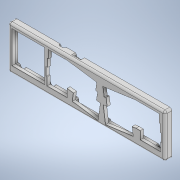
# Autodesk Inventor part: Prime_BLE_Top
Saved by Autodesk Inventor 2020 (Build 240168000, 168)
## iProperties
Created: 2019-06-10
Part Number: Prime_BLE_Top
Material: Generic
Document SubType Name: Modeling
Designer: Holt
Density: 1 g/cm^3
Appearance: Default
Author: Holt
Autodesk Inventor part; units mm, degrees
ref_plane "YZ Plane" through (0, 0, 0) normal (1, 0, 0) x (0, 1, 0)
ref_plane "XZ Plane" through (0, 0, 0) normal (0, 1, 0) x (-1, 0, 0)
ref_plane "XY Plane" through (0, 0, 0) normal (0, 0, 1) x (1, 0, 0)
sketch "Sketch1" plane through (0, 0, 0) normal (0, 0, 1) x (1, 0, 0)
  line L0 (193.827, 71.8136) -> (191.879, 57.9494)
  line L1 (191.879, 57.9494) -> (178.015, 59.8978)
  line L2 (178.015, 59.8978) -> (179.964, 73.7609)
  line L3 (179.964, 73.7609) -> (193.827, 71.8136)
  line L4 (335.021, 71.8149) -> (348.885, 73.7633)
  line L5 (348.885, 73.7633) -> (350.832, 59.8991)
  line L6 (350.832, 59.8991) -> (336.97, 57.9503)
  line L7 (336.97, 57.9503) -> (335.021, 71.8149)
  line L8 (137.682, 59.5644) -> (137.682, 73.5665)
  line L9 (137.682, 73.5665) -> (151.684, 73.5665)
  line L10 (151.684, 73.5665) -> (151.684, 59.5644)
  line L11 (151.684, 59.5644) -> (137.682, 59.5644)
  line L12 (173.018, 59.5644) -> (159.019, 59.5644)
  line L13 (159.019, 59.5644) -> (159.019, 73.5665)
  line L14 (159.019, 73.5665) -> (173.018, 73.5665)
  line L15 (173.018, 73.5665) -> (173.018, 59.5644)
  line L16 (369.901, 73.4147) -> (369.901, 59.4126)
  line L17 (369.901, 59.4126) -> (355.9, 59.4126)
  line L18 (355.9, 59.4126) -> (355.9, 73.4147)
  line L19 (355.9, 73.4147) -> (369.901, 73.4147)
  line L20 (382.093, 59.4126) -> (382.093, 73.4147)
  line L21 (382.093, 73.4147) -> (396.095, 73.4147)
  line L22 (396.095, 73.4147) -> (396.095, 59.4126)
  line L23 (396.095, 59.4126) -> (382.093, 59.4126)
  line L24 (271.059, 82.062) -> (284.924, 84.0118)
  line L25 (284.924, 84.0118) -> (286.872, 70.1473)
  line L26 (286.872, 70.1473) -> (273.008, 68.1989)
  line L27 (273.008, 68.1989) -> (271.059, 82.062)
  line L28 (248.36, 83.3998) -> (246.4211, 69.534)
  line L29 (246.4211, 69.534) -> (232.5558, 71.4724)
  line L30 (232.5558, 71.4724) -> (234.4947, 85.3381)
  line L31 (234.4947, 85.3381) -> (248.36, 83.3998)
  line L32 (291.873, 70.8504) -> (289.925, 84.7135)
  line L33 (289.925, 84.7135) -> (303.788, 86.6619)
  line L34 (303.788, 86.6619) -> (305.736, 72.7988)
  line L35 (305.736, 72.7988) -> (291.873, 70.8504)
  line L36 (227.5465, 72.1776) -> (213.6831, 74.1236)
  line L37 (213.6831, 74.1236) -> (215.6277, 87.9871)
  line L38 (215.6277, 87.9871) -> (229.4921, 86.0411)
  line L39 (229.4921, 86.0411) -> (227.5465, 72.1776)
  line L40 (324.5931, 75.4388) -> (310.7292, 73.498)
  line L41 (310.7292, 73.498) -> (308.7877, 87.3634)
  line L42 (308.7877, 87.3634) -> (322.6526, 89.3043)
  line L43 (322.6526, 89.3043) -> (324.5931, 75.4388)
  line L44 (194.8151, 76.7745) -> (196.7632, 90.6378)
  line L45 (196.7632, 90.6378) -> (210.6263, 88.6898)
  line L46 (210.6263, 88.6898) -> (208.6802, 74.8256)
  line L47 (208.6802, 74.8256) -> (194.8151, 76.7745)
  line L48 (341.5207, 91.9896) -> (343.4929, 78.13)
  line L49 (343.4929, 78.13) -> (329.6334, 76.1573)
  line L50 (329.6334, 76.1573) -> (327.6601, 90.017)
  line L51 (327.6601, 90.017) -> (341.5207, 91.9896)
  line L52 (177.899, 93.2889) -> (191.762, 91.3405)
  line L53 (191.762, 91.3405) -> (189.814, 77.4774)
  line L54 (189.814, 77.4774) -> (175.949, 79.4247)
  line L55 (175.949, 79.4247) -> (177.899, 93.2889)
  line L56 (367.52, 78.6542) -> (367.52, 92.6549)
  line L57 (367.52, 92.6549) -> (381.52, 92.6549)
  line L58 (381.52, 92.6549) -> (381.52, 78.6542)
  line L59 (381.52, 78.6542) -> (367.52, 78.6542)
  line L60 (400.572, 92.6549) -> (400.572, 78.6542)
  line L61 (400.572, 78.6542) -> (386.572, 78.6542)
  line L62 (386.572, 78.6542) -> (386.572, 92.6549)
  line L63 (386.572, 92.6549) -> (400.572, 92.6549)
  line L64 (151.874, 78.8046) -> (137.874, 78.8046)
  line L65 (137.874, 78.8046) -> (137.874, 92.8067)
  line L66 (137.874, 92.8067) -> (151.874, 92.8067)
  line L67 (151.874, 92.8067) -> (151.874, 78.8046)
  line L68 (156.924, 92.8067) -> (170.924, 92.8067)
  line L69 (170.924, 92.8067) -> (170.924, 78.8046)
  line L70 (170.924, 78.8046) -> (156.924, 78.8046)
  line L71 (156.924, 78.8046) -> (156.924, 92.8067)
  line L72 (348.47, 78.6528) -> (348.47, 92.6549)
  line L73 (348.47, 92.6549) -> (362.472, 92.6549)
  line L74 (362.472, 92.6549) -> (362.472, 78.6528)
  line L75 (362.472, 78.6528) -> (348.47, 78.6528)
  line L76 (279.4658, 26.5127) -> (282.7331, 26.9708)
  line L77 (282.7331, 26.9708) -> (282.8681, 26.0103)
  line L78 (282.8681, 26.0103) -> (303.1679, 28.8637)
  line L79 (303.1679, 28.8637) -> (303.033, 29.8243)
  line L80 (303.033, 29.8243) -> (306.3022, 30.2828)
  line L81 (306.3022, 30.2828) -> (306.4372, 29.3223)
  line L82 (306.4372, 29.3223) -> (309.383, 29.737)
  line L83 (309.383, 29.737) -> (311.3317, 15.874)
  line L84 (311.3317, 15.874) -> (278.603, 11.273)
  line L85 (278.603, 11.273) -> (276.6549, 25.1376)
  line L86 (276.6549, 25.1376) -> (279.6011, 25.5509)
  line L87 (279.6011, 25.5509) -> (279.4658, 26.5127)
  line L88 (106.443, 78.8067) -> (106.443, 92.8067)
  line L89 (106.443, 92.8067) -> (120.443, 92.8067)
  line L90 (120.443, 92.8067) -> (120.443, 78.8067)
  line L91 (120.443, 78.8067) -> (106.443, 78.8067)
  line L92 (101.393, 78.8067) -> (87.393, 78.8067)
  line L93 (87.393, 78.8067) -> (87.393, 92.8067)
  line L94 (87.393, 92.8067) -> (101.393, 92.8067)
  line L95 (101.393, 92.8067) -> (101.393, 78.8067)
  line L96 (68.343, 92.8067) -> (82.343, 92.8067)
  line L97 (82.343, 92.8067) -> (82.343, 78.8067)
  line L98 (82.343, 78.8067) -> (68.343, 78.8067)
  line L99 (68.343, 78.8067) -> (68.343, 92.8067)
  line L100 (49.293, 78.8067) -> (49.293, 92.8067)
  line L101 (49.293, 92.8067) -> (63.293, 92.8067)
  line L102 (63.293, 92.8067) -> (63.293, 78.8067)
  line L103 (63.293, 78.8067) -> (49.293, 78.8067)
  line L104 (120.443, 59.7567) -> (106.443, 59.7567)
  line L105 (106.443, 59.7567) -> (106.443, 73.7567)
  line L106 (106.443, 73.7567) -> (120.443, 73.7567)
  line L107 (120.443, 73.7567) -> (120.443, 59.7567)
  line L108 (87.393, 59.7567) -> (87.393, 73.7567)
  line L109 (87.393, 73.7567) -> (101.393, 73.7567)
  line L110 (101.393, 73.7567) -> (101.393, 59.7567)
  line L111 (101.393, 59.7567) -> (87.393, 59.7567)
  line L112 (68.343, 73.7567) -> (82.343, 73.7567)
  line L113 (82.343, 73.7567) -> (82.343, 59.7567)
  line L114 (82.343, 59.7567) -> (68.343, 59.7567)
  line L115 (68.343, 59.7567) -> (68.343, 73.7567)
  line L116 (63.293, 73.7567) -> (63.293, 59.7567)
  line L117 (63.293, 59.7567) -> (49.293, 59.7567)
  line L118 (49.293, 59.7567) -> (49.293, 73.7567)
  line L119 (49.293, 73.7567) -> (63.293, 73.7567)
  line L120 (106.443, 54.7067) -> (120.443, 54.7067)
  line L121 (120.443, 54.7067) -> (120.443, 40.7067)
  line L122 (120.443, 40.7067) -> (106.443, 40.7067)
  line L123 (106.443, 40.7067) -> (106.443, 54.7067)
  line L124 (101.393, 40.7067) -> (87.393, 40.7067)
  line L125 (87.393, 40.7067) -> (87.393, 54.7067)
  line L126 (87.393, 54.7067) -> (101.393, 54.7067)
  line L127 (101.393, 54.7067) -> (101.393, 40.7067)
  line L128 (68.343, 54.7067) -> (82.343, 54.7067)
  line L129 (82.343, 54.7067) -> (82.343, 40.7067)
  line L130 (82.343, 40.7067) -> (68.343, 40.7067)
  line L131 (68.343, 40.7067) -> (68.343, 54.7067)
  line L132 (63.293, 40.7067) -> (49.293, 40.7067)
  line L133 (49.293, 40.7067) -> (49.293, 54.7067)
  line L134 (49.293, 54.7067) -> (63.293, 54.7067)
  line L135 (63.293, 54.7067) -> (63.293, 40.7067)
  line L136 (120.443, 35.6567) -> (120.443, 21.6567)
  line L137 (120.443, 21.6567) -> (106.443, 21.6567)
  line L138 (106.443, 21.6567) -> (106.443, 35.6567)
  line L139 (106.443, 35.6567) -> (120.443, 35.6567)
  line L140 (101.393, 35.6567) -> (101.393, 21.6567)
  line L141 (101.393, 21.6567) -> (87.393, 21.6567)
  line L142 (87.393, 21.6567) -> (87.393, 35.6567)
  line L143 (87.393, 35.6567) -> (101.393, 35.6567)
  line L144 (82.343, 35.6567) -> (82.343, 21.6567)
  line L145 (82.343, 21.6567) -> (68.343, 21.6567)
  line L146 (68.343, 21.6567) -> (68.343, 35.6567)
  line L147 (68.343, 35.6567) -> (82.343, 35.6567)
  line L148 (49.293, 35.6567) -> (63.293, 35.6567)
  line L149 (63.293, 35.6567) -> (63.293, 21.6567)
  line L150 (63.293, 21.6567) -> (49.293, 21.6567)
  line L151 (49.293, 21.6567) -> (49.293, 35.6567)
  line L152 (214.464, 30.4381) -> (212.514, 16.5751)
  line L153 (212.514, 16.5751) -> (198.651, 18.5236)
  line L154 (198.651, 18.5236) -> (200.6, 32.3867)
  line L155 (200.6, 32.3867) -> (214.464, 30.4381)
  line L156 (254.551, 24.8047) -> (252.603, 10.9416)
  line L157 (252.603, 10.9416) -> (219.874, 15.5401)
  line L158 (219.874, 15.5401) -> (221.823, 29.4046)
  line L159 (221.823, 29.4046) -> (224.769, 28.9898)
  line L160 (224.769, 28.9898) -> (224.904, 29.9516)
  line L161 (224.904, 29.9516) -> (228.171, 29.4914)
  line L162 (228.171, 29.4914) -> (228.036, 28.5309)
  line L163 (228.036, 28.5309) -> (248.336, 25.6784)
  line L164 (248.336, 25.6784) -> (248.471, 26.6389)
  line L165 (248.471, 26.6389) -> (251.74, 26.1786)
  line L166 (251.74, 26.1786) -> (251.605, 25.2181)
  line L167 (251.605, 25.2181) -> (254.551, 24.8047)
  line L168 (150.826, 35.0848) -> (150.826, 21.0854)
  line L169 (150.826, 21.0854) -> (136.826, 21.0854)
  line L170 (136.826, 21.0854) -> (136.826, 35.0848)
  line L171 (136.826, 35.0848) -> (150.826, 35.0848)
  line L172 (160.638, 35.0848) -> (174.637, 35.0848)
  line L173 (174.637, 35.0848) -> (174.637, 21.0854)
  line L174 (174.637, 21.0854) -> (160.638, 21.0854)
  line L175 (160.638, 21.0854) -> (160.638, 35.0848)
  line L176 (334.913, 19.1876) -> (321.049, 17.2391)
  line L177 (321.049, 17.2391) -> (319.1, 31.1021)
  line L178 (319.1, 31.1021) -> (332.965, 33.052)
  line L179 (332.965, 33.052) -> (334.913, 19.1876)
  line L180 (387.427, 20.9336) -> (387.427, 34.933)
  line L181 (387.427, 34.933) -> (401.426, 34.933)
  line L182 (401.426, 34.933) -> (401.426, 20.9336)
  line L183 (401.426, 20.9336) -> (387.427, 20.9336)
  line L184 (271.646, 43.6699) -> (285.509, 45.6197)
  line L185 (285.509, 45.6197) -> (287.459, 31.7553)
  line L186 (287.459, 31.7553) -> (273.595, 29.8068)
  line L187 (273.595, 29.8068) -> (271.646, 43.6699)
  line L188 (377.617, 34.933) -> (377.617, 20.9336)
  line L189 (377.617, 20.9336) -> (363.615, 20.9336)
  line L190 (363.615, 20.9336) -> (363.615, 34.933)
  line L191 (363.615, 34.933) -> (377.617, 34.933)
  line L192 (224.474, 48.2685) -> (238.337, 46.3201)
  line L193 (238.337, 46.3201) -> (236.389, 32.4569)
  line L194 (236.389, 32.4569) -> (222.526, 34.4055)
  line L195 (222.526, 34.4055) -> (224.474, 48.2685)
  line L196 (255.254, 29.8056) -> (241.39, 31.7541)
  line L197 (241.39, 31.7541) -> (243.338, 45.6188)
  line L198 (243.338, 45.6188) -> (257.201, 43.6686)
  line L199 (257.201, 43.6686) -> (255.254, 29.8056)
  line L200 (200.609, 51.6227) -> (198.659, 37.7596)
  line L201 (198.659, 37.7596) -> (184.796, 39.7083)
  line L202 (184.796, 39.7083) -> (186.745, 53.5711)
  line L203 (186.745, 53.5711) -> (200.609, 51.6227)
  line L204 (342.104, 53.5724) -> (344.051, 39.7093)
  line L205 (344.051, 39.7093) -> (330.188, 37.7609)
  line L206 (330.188, 37.7609) -> (328.239, 51.624)
  line L207 (328.239, 51.624) -> (342.104, 53.5724)
  line L208 (292.459, 32.4581) -> (290.51, 46.321)
  line L209 (290.51, 46.321) -> (304.375, 48.2712)
  line L210 (304.375, 48.2712) -> (306.323, 34.4066)
  line L211 (306.323, 34.4066) -> (292.459, 32.4581)
  line L212 (139.493, 54.325) -> (153.493, 54.325)
  line L213 (153.493, 54.325) -> (153.493, 40.3243)
  line L214 (153.493, 40.3243) -> (139.493, 40.3243)
  line L215 (139.493, 40.3243) -> (139.493, 54.325)
  line L216 (179.687, 54.325) -> (179.687, 40.3243)
  line L217 (179.687, 40.3243) -> (165.687, 40.3243)
  line L218 (165.687, 40.3243) -> (165.687, 54.325)
  line L219 (165.687, 54.325) -> (179.687, 54.325)
  line L220 (219.473, 48.9726) -> (217.525, 35.1083)
  line L221 (217.525, 35.1083) -> (203.66, 37.0568)
  line L222 (203.66, 37.0568) -> (205.609, 50.9199)
  line L223 (205.609, 50.9199) -> (219.473, 48.9726)
  line L224 (309.376, 48.9739) -> (323.239, 50.9209)
  line L225 (323.239, 50.9209) -> (325.187, 37.0581)
  line L226 (325.187, 37.0581) -> (311.324, 35.1094)
  line L227 (311.324, 35.1094) -> (309.376, 48.9739)
  line L228 (382.093, 40.1725) -> (368.092, 40.1725)
  line L229 (368.092, 40.1725) -> (368.092, 54.1732)
  line L230 (368.092, 54.1732) -> (382.093, 54.1732)
  line L231 (382.093, 54.1732) -> (382.093, 40.1725)
  line L232 (389.523, 40.1725) -> (389.523, 54.1732)
  line L233 (389.523, 54.1732) -> (403.525, 54.1732)
  line L234 (403.525, 54.1732) -> (403.525, 40.1725)
  line L235 (403.525, 40.1725) -> (389.523, 40.1725)
  line L236 (250.421, 63.8598) -> (248.473, 49.9967)
  line L237 (248.473, 49.9967) -> (234.608, 51.9437)
  line L238 (234.608, 51.9437) -> (236.558, 65.8082)
  line L239 (236.558, 65.8082) -> (250.421, 63.8598)
  line L240 (278.426, 63.8608) -> (292.291, 65.8095)
  line L241 (292.291, 65.8095) -> (294.239, 51.945)
  line L242 (294.239, 51.945) -> (280.376, 49.9977)
  line L243 (280.376, 49.9977) -> (278.426, 63.8608)
  line L244 (229.607, 52.6464) -> (215.744, 54.5952)
  line L245 (215.744, 54.5952) -> (217.693, 68.4597)
  line L246 (217.693, 68.4597) -> (231.557, 66.511)
  line L247 (231.557, 66.511) -> (229.607, 52.6464)
  line L248 (299.24, 52.6477) -> (297.292, 66.5123)
  line L249 (297.292, 66.5123) -> (311.156, 68.4607)
  line L250 (311.156, 68.4607) -> (313.103, 54.5961)
  line L251 (313.103, 54.5961) -> (299.24, 52.6477)
  line L252 (363.043, 40.1725) -> (349.042, 40.1725)
  line L253 (349.042, 40.1725) -> (349.042, 54.1732)
  line L254 (349.042, 54.1732) -> (363.043, 54.1732)
  line L255 (363.043, 54.1732) -> (363.043, 40.1725)
  line L256 (198.827, 71.1094) -> (212.692, 69.1624)
  line L257 (212.692, 69.1624) -> (210.743, 55.2979)
  line L258 (210.743, 55.2979) -> (196.88, 57.2463)
  line L259 (196.88, 57.2463) -> (198.827, 71.1094)
  line L260 (331.969, 57.249) -> (318.105, 55.2992)
  line L261 (318.105, 55.2992) -> (316.157, 69.1634)
  line L262 (316.157, 69.1634) -> (330.02, 71.1121)
  line L263 (330.02, 71.1121) -> (331.969, 57.249)
  point P0 (0, 0)
  constraints: 528 end point
sketch "Sketch2" plane through (0, 0, 0) normal (0, 0, 1) x (1, 0, 0)
  line L0 (46.218, 95.8817) -> (46.218, 18.0104)
  line L1 (49.293, 59.7567) -> (49.293, 73.7567) projected
  line L2 (101.393, 21.6567) -> (87.393, 21.6567) projected
  line L3 (150.826, 21.0854) -> (136.826, 21.0854) projected
  line L4 (212.514, 16.5751) -> (198.651, 18.5236) projected
  line L5 (311.3317, 15.874) -> (278.603, 11.273) projected
  line L6 (377.617, 20.9336) -> (363.615, 20.9336) projected
  line L7 (401.426, 34.933) -> (401.426, 20.9336) projected
  line L8 (403.525, 54.1732) -> (403.525, 40.1725) projected
  line L9 (396.095, 73.4147) -> (396.095, 59.4126) projected
  line L10 (400.572, 92.6549) -> (400.572, 78.6542) projected
  line L11 (386.572, 92.6549) -> (400.572, 92.6549) projected
  line L12 (271.059, 82.062) -> (284.924, 84.0118) projected
  line L13 (234.4947, 85.3381) -> (248.36, 83.3998) projected
  line L14 (250.421, 63.8598) -> (248.473, 49.9967) projected
  line L15 (257.201, 43.6686) -> (255.254, 29.8056) projected
  line L16 (273.595, 29.8068) -> (271.646, 43.6699) projected
  line L17 (254.551, 24.8047) -> (252.603, 10.9416) projected
  line L18 (278.603, 11.273) -> (276.6549, 25.1376) projected
  line L19 (280.376, 49.9977) -> (278.426, 63.8608) projected
  line L20 (273.008, 68.1989) -> (271.059, 82.062) projected
  line L21 (49.293, 92.8067) -> (63.293, 92.8067) projected
  line L22 (137.874, 92.8067) -> (151.874, 92.8067) projected
  line L23 (177.899, 93.2889) -> (191.762, 91.3405) projected
  line L24 (175.949, 79.4247) -> (177.899, 93.2889) projected
  line L25 (175.2822, 96.7619) -> (181.5449, 95.8817)
  line L26 (175.1584, 95.8817) -> (175.2822, 96.7619)
  line L27 (192.82, 16.2379) -> (255.22, 7.4674)
  line L28 (253.5963, 18.0104) -> (253.5974, 18.0104)
  line L29 (124.6706, 95.8817) -> (124.6706, 18.0104)
  line L30 (120.443, 73.7567) -> (120.443, 59.7567) projected
  line L31 (137.874, 78.8046) -> (137.874, 92.8067) projected
  line L32 (137.682, 59.5644) -> (137.682, 73.5665) projected
  line L33 (139.493, 40.3243) -> (139.493, 54.325) projected
  line L34 (136.826, 21.0854) -> (136.826, 35.0848) projected
  line L35 (248.36, 83.3998) -> (246.4211, 69.534) projected
  line L36 (251.829, 86.0035) -> (249.1909, 67.1379)
  line L37 (253.4661, 63.4319) -> (251.2431, 47.612)
  line L38 (269.9629, 67.7708) -> (267.5859, 84.6788)
  line L39 (277.6061, 47.6134) -> (275.1058, 65.3885)
  line L40 (273.6303, 7.4687) -> (268.1729, 46.2867)
  line L41 (243.338, 45.6188) -> (257.201, 43.6686) projected
  line L42 (236.558, 65.8082) -> (250.421, 63.8598) projected
  line L43 (286.872, 70.1473) -> (273.008, 68.1989) projected
  line L44 (271.646, 43.6699) -> (285.509, 45.6197) projected
  line L45 (275.1058, 65.3885) -> (273.4359, 65.1538)
  line L46 (271.2177, 46.7149) -> (277.6061, 47.6134)
  line L47 (181.5449, 95.8817) -> (251.829, 86.0035)
  line L48 (346.1698, 95.7299) -> (267.5859, 84.6788)
  line L49 (253.894, 66.4769) -> (253.4661, 63.4319)
  line L50 (271.2177, 46.7149) -> (268.1729, 46.2867)
  line L51 (269.9629, 67.7708) -> (270.391, 64.7257)
  line L52 (270.391, 64.7257) -> (273.4359, 65.1538)
  line L53 (406.882, 17.8586) -> (358.159, 17.8586)
  line L54 (340.7435, 16.9034) -> (273.6303, 7.4687)
  line L55 (403.647, 95.8817) -> (403.647, 76.4897)
  line L56 (406.314, 73.4147) -> (406.314, 57.2482)
  line L57 (408.981, 54.1732) -> (408.981, 40.1725)
  line L58 (406.882, 37.0975) -> (406.882, 17.8586)
  line L59 (131.37, 18.0104) -> (131.37, 37.2493)
  line L60 (132.226, 57.4) -> (132.226, 73.5665)
  line L61 (134.799, 76.6415) -> (134.799, 95.8817)
  line L62 (129.274, 40.3243) -> (129.274, 54.325)
  line L63 (153.493, 40.3243) -> (139.493, 40.3243) projected
  line L64 (139.493, 54.325) -> (153.493, 54.325) projected
  line L65 (137.682, 73.5665) -> (151.684, 73.5665) projected
  line L66 (403.525, 40.1725) -> (389.523, 40.1725) projected
  line L67 (389.523, 54.1732) -> (403.525, 54.1732) projected
  line L68 (382.093, 73.4147) -> (396.095, 73.4147) projected
  line L69 (174.637, 35.0848) -> (174.637, 21.0854) projected
  line L70 (198.651, 18.5236) -> (200.6, 32.3867) projected
  line L71 (198.659, 37.7596) -> (184.796, 39.7083) projected
  line L72 (179.687, 40.3243) -> (165.687, 40.3243) projected
  line L73 (332.965, 33.052) -> (334.913, 19.1876) projected
  line L74 (344.051, 39.7093) -> (330.188, 37.7609) projected
  line L75 (363.043, 40.1725) -> (349.042, 40.1725) projected
  line L76 (363.615, 20.9336) -> (363.615, 34.933) projected
  line L77 (192.82, 16.2379) -> (195.4721, 35.1023)
  line L78 (180.093, 37.2493) -> (180.093, 18.0104)
  line L79 (195.4721, 35.1023) -> (180.1987, 37.2493)
  line L80 (338.0932, 35.7667) -> (340.7435, 16.9034)
  line L81 (358.159, 17.8586) -> (358.159, 37.0975)
  line L82 (344.479, 36.6642) -> (338.0932, 35.7667)
  line L83 (358.159, 37.0975) -> (347.5617, 37.0975)
  line L84 (344.479, 36.6642) -> (347.5617, 37.0975)
  line L85 (180.093, 37.2493) -> (180.1987, 37.2493)
  line L86 (408.981, 40.1725) -> (408.981, 37.0975)
  line L87 (408.981, 37.0975) -> (406.882, 37.0975)
  line L88 (408.981, 54.1732) -> (408.981, 57.2482)
  line L89 (408.981, 57.2482) -> (406.314, 57.2482)
  line L90 (406.314, 73.4147) -> (406.314, 76.4897)
  line L91 (406.314, 76.4897) -> (403.647, 76.4897)
  line L92 (131.37, 37.2493) -> (129.274, 37.2493)
  line L93 (129.274, 37.2493) -> (129.274, 40.3243)
  line L94 (132.226, 57.4) -> (129.274, 57.4)
  line L95 (129.274, 57.4) -> (129.274, 54.325)
  line L96 (134.799, 76.6415) -> (132.226, 76.6415)
  line L97 (132.226, 76.6415) -> (132.226, 73.5665)
  line L98 (46.218, 95.8817) -> (124.6706, 95.8817)
  line L99 (134.799, 95.8817) -> (175.1584, 95.8817)
  line L100 (46.218, 18.0104) -> (124.6706, 18.0104)
  line L101 (131.37, 18.0104) -> (180.2095, 18.0104)
  line L102 (346.1698, 95.7299) -> (403.647, 95.7299)
  line L103 (255.22, 7.4674) -> (260.674, 46.2858)
  line L104 (251.2431, 47.612) -> (260.674, 46.2858)
  line L105 (249.1909, 67.1379) -> (253.894, 66.4769)
  line L106 (416.518, 103.2669) -> (38.681, 103.2669)
  line L107 (38.681, 103.2669) -> (38.681, 10.4734)
  line L108 (38.681, 10.4734) -> (124.6706, 10.4734)
  line L109 (124.6706, 10.4734) -> (131.37, 10.4734)
  line L110 (131.37, 10.4734) -> (179.6824, 10.4734)
  line L111 (348.0651, 10.3216) -> (358.159, 10.3216)
  line L112 (358.159, 10.3216) -> (416.518, 10.3216)
  line L113 (416.518, 10.3216) -> (416.518, 103.2669)
  line L114 (348.0651, 10.3216) -> (348.0651, -1.6784)
  line L115 (348.0651, -1.6784) -> (179.6824, -1.6784)
  line L116 (179.6824, -1.6784) -> (179.6824, 10.4734)
  point P0 (0, 0)
  dimension "d1" = 3.075
  dimension "d5" = 3.075
  dimension "d7" = 3.075
  dimension "d8" = 4.2276
  dimension "d9" = 3.075
  dimension "d10" = 3.075
  dimension "d12" = 3.075
  dimension "d13" = 3.075
  dimension "d14" = 3.075
  dimension "d18" = 3.075
  dimension "d19" = 3.075
  dimension "d22" = 3.075
  dimension "d23" = 3.075
  dimension "d24" = 10.219
  dimension "d25" = 5.456
  dimension "d26" = 5.456
  dimension "d27" = 5.456
  dimension "d28" = 5.456
  dimension "d29" = 3.075
  dimension "d30" = 10.219
  dimension "d37" = 5.456
  dimension "d38" = 5.456
  dimension "d39" = 3.075
  dimension "d41" = 5.456
  dimension "d42" = 5.456
  dimension "d43" = 3.075
  dimension "d44" = 3.075
  dimension "d61" = 12
  constraints: 138 end point, 29 parallel, 10 perpendicular, 8 horizontal, 6 point on line, 5 vertical, 4 collinear
  measures "d1" distance between parallel lines of L0 L1
  measures "d5" distance between parallel lines of L23 L25
  measures "d7" distance between parallel lines of L27 L4
  measures "d8" distance between parallel lines of L29 L30
  measures "d9" distance between parallel lines of L35 L36
  measures "d10" distance between parallel lines of L14 L37
  measures "d12" distance between parallel lines of L20 L38
  measures "d13" distance between parallel lines of L19 L39
  measures "d14" distance between parallel lines of L16 L40
  measures "d18" distance between parallel lines of L43 L45
  measures "d19" distance between parallel lines of L44 L46
  measures "d22" distance between parallel lines of L53 L6
  measures "d23" distance between parallel lines of L10 L55
  measures "d24" distance between parallel lines of L9 L56
  measures "d25" distance between parallel lines of L8 L57
  measures "d26" distance between parallel lines of L7 L58
  measures "d27" distance between parallel lines of L34 L59
  measures "d28" distance between parallel lines of L32 L60
  measures "d29" distance between parallel lines of L31 L61
  measures "d30" distance between parallel lines of L33 L62
  measures "d37" distance between parallel lines of L70 L77
  measures "d38" distance between parallel lines of L69 L78
  measures "d39" distance between parallel lines of L71 L79
  measures "d41" distance between parallel lines of L73 L80
  measures "d42" distance between parallel lines of L76 L81
  measures "d43" distance between parallel lines of L74 L82
  measures "d44" distance between parallel lines of L75 L83
  measures "d61" distance of L111.start L114.end
extrude "Extrusion3" add sketch "Sketch2" along normal blind 7.65
sketch "Sketch3" plane through (0, 0, 0) normal (0, 0, -1) x (-1, 0, 0)
  line L0 (-348.0651, 10.3216) -> (-416.518, 10.3216) projected
  line L1 (-348.0651, -1.6784) -> (-348.0651, 10.3216) projected
  line L2 (-179.6824, -1.6784) -> (-348.0651, -1.6784) projected
  line L3 (-179.6824, 10.4734) -> (-179.6824, -1.6784) projected
  line L4 (-38.681, 10.4734) -> (-179.6824, 10.4734) projected
  line L5 (-38.681, 103.2669) -> (-38.681, 10.4734) projected
  line L6 (-416.518, 103.2669) -> (-38.681, 103.2669) projected
  line L7 (-416.518, 10.3216) -> (-416.518, 103.2669) projected
  line L8 (-124.6706, 18.0104) -> (-46.218, 18.0104) projected
  line L9 (-124.6706, 95.8817) -> (-124.6706, 18.0104) projected
  line L10 (-46.218, 95.8817) -> (-124.6706, 95.8817) projected
  line L11 (-46.218, 18.0104) -> (-46.218, 95.8817) projected
  line L12 (-268.1729, 46.2867) -> (-277.6061, 47.6134) projected
  line L13 (-273.6303, 7.4687) -> (-268.1729, 46.2867) projected
  line L14 (-340.7435, 16.9034) -> (-273.6303, 7.4687) projected
  line L15 (-338.0932, 35.7667) -> (-340.7435, 16.9034) projected
  line L16 (-347.5617, 37.0975) -> (-338.0932, 35.7667) projected
  line L17 (-358.159, 37.0975) -> (-347.5617, 37.0975) projected
  line L18 (-358.159, 17.8586) -> (-358.159, 37.0975) projected
  line L19 (-406.882, 17.8586) -> (-358.159, 17.8586) projected
  line L20 (-406.882, 37.0975) -> (-406.882, 17.8586) projected
  line L21 (-408.981, 37.0975) -> (-406.882, 37.0975) projected
  line L22 (-408.981, 57.2482) -> (-408.981, 37.0975) projected
  line L23 (-406.314, 57.2482) -> (-408.981, 57.2482) projected
  line L24 (-406.314, 76.4897) -> (-406.314, 57.2482) projected
  line L25 (-403.647, 76.4897) -> (-406.314, 76.4897) projected
  line L26 (-403.647, 95.7299) -> (-403.647, 76.4897) projected
  line L27 (-346.1698, 95.7299) -> (-403.647, 95.7299) projected
  line L28 (-267.5859, 84.6788) -> (-346.1698, 95.7299) projected
  line L29 (-270.391, 64.7257) -> (-267.5859, 84.6788) projected
  line L30 (-273.4359, 65.1538) -> (-270.391, 64.7257) projected
  line L31 (-275.1058, 65.3885) -> (-273.4359, 65.1538) projected
  line L32 (-277.6061, 47.6134) -> (-275.1058, 65.3885) projected
  line L33 (-132.226, 57.4) -> (-132.226, 76.6415) projected
  line L34 (-129.274, 57.4) -> (-132.226, 57.4) projected
  line L35 (-129.274, 37.2493) -> (-129.274, 57.4) projected
  line L36 (-131.37, 37.2493) -> (-129.274, 37.2493) projected
  line L37 (-131.37, 18.0104) -> (-131.37, 37.2493) projected
  line L38 (-180.093, 18.0104) -> (-131.37, 18.0104) projected
  line L39 (-180.093, 37.2493) -> (-180.093, 18.0104) projected
  line L40 (-180.1987, 37.2493) -> (-180.093, 37.2493) projected
  line L41 (-195.4721, 35.1023) -> (-180.1987, 37.2493) projected
  line L42 (-192.82, 16.2379) -> (-195.4721, 35.1023) projected
  line L43 (-255.22, 7.4674) -> (-192.82, 16.2379) projected
  line L44 (-260.674, 46.2858) -> (-255.22, 7.4674) projected
  line L45 (-251.2431, 47.612) -> (-260.674, 46.2858) projected
  line L46 (-253.894, 66.4769) -> (-251.2431, 47.612) projected
  line L47 (-249.1909, 67.1379) -> (-253.894, 66.4769) projected
  line L48 (-251.829, 86.0035) -> (-249.1909, 67.1379) projected
  line L49 (-175.2822, 96.7619) -> (-251.829, 86.0035) projected
  line L50 (-175.1584, 95.8817) -> (-175.2822, 96.7619) projected
  line L51 (-134.799, 95.8817) -> (-175.1584, 95.8817) projected
  line L52 (-134.799, 76.6415) -> (-134.799, 95.8817) projected
  line L53 (-132.226, 76.6415) -> (-134.799, 76.6415) projected
  line L54 (-343.0651, 3.3216) -> (-343.0651, 15.3216)
  line L55 (-343.0651, 15.3216) -> (-411.518, 15.3216)
  line L56 (-411.518, 15.3216) -> (-411.518, 98.2669)
  line L57 (-411.518, 98.2669) -> (-43.681, 98.2669)
  line L58 (-43.681, 98.2669) -> (-43.681, 15.4734)
  line L59 (-43.681, 15.4734) -> (-184.6824, 15.4734)
  line L60 (-184.6824, 15.4734) -> (-184.6824, 3.3216)
  line L61 (-184.6824, 3.3216) -> (-343.0651, 3.3216)
  point P0 (0, 0)
  dimension "d62" = 5
  constraints: 16 end point, 7 other
  measures "d62" distance between parallel lines of L2 L61
extrude "Extrusion4" add sketch "Sketch3" along normal blind 8.255 contours L0 L7 L6 L5 L4 L3 L2 L1
sketch "Sketch4" plane through (0, 0, -8.255) normal (0, 0, -1) x (-1, 0, 0)
  line L0 (-38.681, 103.2669) -> (-416.518, 103.2669) projected
  line L1 (-411.518, 98.2669) -> (-43.681, 98.2669) projected
  line L2 (-159.963, 103.2669) -> (-148.963, 103.2669)
  line L3 (-148.963, 103.2669) -> (-148.963, 98.2669)
  line L4 (-148.963, 98.2669) -> (-159.963, 98.2669)
  line L5 (-159.963, 98.2669) -> (-159.963, 103.2669)
  line L6 (-38.681, 10.4734) -> (-38.681, 103.2669) projected
  point P0 (0, 0)
  point P1 (-159.963, 98.2669)
  dimension "d65" = 11
  dimension "d66" = 110.282
  constraints: 8 end point, 2 parallel, 2 point on line, 1 horizontal, 1 perpendicular
  measures "d65" distance of L3.end L4.end
  measures "d66" distance between parallel lines of L3 L6
extrude "Extrusion5" cut sketch "Sketch4" against normal blind 4
sketch "Sketch5" plane through (0, 0, -4.255) normal (0, 0, -1) x (-1, 0, 0)
  line L0 (-159.963, 98.2669) -> (-159.963, 103.2669) projected
  line L1 (-148.963, 103.2669) -> (-148.963, 98.2669) projected
  line L2 (-159.963, 103.2669) -> (-148.963, 103.2669)
  line L3 (-148.963, 103.2669) -> (-148.963, 102.2669)
  line L4 (-148.963, 102.2669) -> (-159.963, 102.2669)
  line L5 (-159.963, 102.2669) -> (-159.963, 103.2669)
  point P0 (0, 0)
  dimension "d69" = 1
  constraints: 8 end point, 2 parallel, 1 horizontal, 1 perpendicular, 1 point on line
  measures "d69" distance of L2.end L3.end
extrude "Extrusion6" add sketch "Sketch5" along normal blind 1.75
sketch "Sketch6" plane through (0, 0, -8.255) normal (0, 0, -1) x (-1, 0, 0)
  line L0 (-413.5189, 98.2669) -> (-413.5189, 60.7669)
  line L1 (-411.518, 98.2669) -> (-411.518, 15.3216) projected
  line L2 (-413.5189, 98.2669) -> (-411.518, 98.2669)
  line L3 (-413.5189, 60.7669) -> (-411.518, 60.7669)
  point P0 (0, 0)
  dimension "d72" = 37.5
  constraints: 6 end point, 1 horizontal, 1 perpendicular, 1 point on line, 1 vertical
  measures "d72" distance of L0.start L0.end
extrude "Extrusion7" cut sketch "Sketch6" against normal up to surface (8.255 mm away)
fillet "Fillet1" radius 2 2 edges at (159.963, 102.7669, -6.005) (148.963, 102.7669, -6.005)
move faces "Move1" translate (7.039, 0, 0) faces at (184.6824, 11.4228, -2.7517)
move faces "Move2" translate (7.039, 0, 0) faces at (179.6824, 2.3722, -0.2017)
move faces "Move3" translate (0, 2.352, 0) faces at (242.1693, 3.3216, -2.7517)
move faces "Move4" translate (0, 2.352, 0) faces at (240.5026, -1.6784, -2.9533)
sketch "Sketch7" plane through (0, 0, -8.255) normal (0, 0, -1) x (-1, 0, 0)
  line L0 (-413.5189, 98.2669) -> (-159.963, 98.2669) projected
  line L1 (-159.963, 102.2669) -> (-161.963, 102.2669)
  line L2 (-161.963, 102.2669) -> (-161.963, 98.2669)
  line L3 (-161.963, 98.2669) -> (-159.963, 98.2669)
  line L4 (-159.963, 98.2669) -> (-159.963, 102.2669)
  line L5 (-148.963, 98.2669) -> (-43.681, 98.2669) projected
  line L6 (-148.963, 102.2669) -> (-146.963, 102.2669)
  line L7 (-146.963, 102.2669) -> (-146.963, 98.2669)
  line L8 (-146.963, 98.2669) -> (-148.963, 98.2669)
  line L9 (-148.963, 98.2669) -> (-148.963, 102.2669)
  point P0 (0, 0)
  point P1 (-159.963, 98.2669)
  dimension "d88" = 2
  dimension "d89" = 2
  constraints: 16 end point, 4 parallel, 2 horizontal, 2 perpendicular, 2 point on line
  measures "d88" distance of L3.end L2.end
  measures "d89" distance of L7.end L8.end
extrude "Extrusion8" cut sketch "Sketch7" against normal up to surface (4 mm away)
move faces "Move5" translate (68.4529, 0, 0) faces at (348.0651, 3.8896, -0.2017)
sketch "Sketch8" plane through (186.7214, 10.4734, -8.255) normal (-1, 0, 0) x (0, 0, 1)
  line L0 (0, -9.7998) -> (15.905, -9.7998) projected
  line L1 (15.905, 0) -> (15.905, -9.7998) projected
  line L2 (0, 0) -> (15.905, 0) projected
  line L3 (0, -9.7998) -> (0, 0) projected
  point P0 (8.255, -10.4734)
extrude "Extrusion9" add sketch "Sketch8" along normal up to surface (148.0404 mm away)
move faces "Move6" translate (0, 3, 0) faces at (202.054, 103.2669, 3.0983)
sketch "Sketch9" plane through (0, 0, -8.255) normal (0, 0, -1) x (-1, 0, 0)
  circle A0 centre (-393.5699, 99.1106) radius 6
  line L0 (-343.0651, 15.3216) -> (-411.518, 15.3216) projected
  line L1 (-413.5189, 60.7669) -> (-413.5189, 98.2669) projected
  circle A1 centre (-258.7819, 99.2406) radius 6
  line L2 (-191.7214, 5.6736) -> (-343.0651, 5.6736) projected
  circle A2 centre (-129.159, 99.3064) radius 6
  line L3 (-43.681, 98.2669) -> (-43.681, 15.4734) projected
  line L4 (-43.681, 15.4734) -> (-191.7214, 15.4734) projected
  circle A3 centre (-56.293, 99.3064) radius 6
  circle A4 centre (-394.426, 14.4339) radius 6
  line L5 (-411.518, 15.3216) -> (-411.518, 60.7669) projected
  line L6 (-413.5189, 98.2669) -> (-161.963, 98.2669) projected
  circle A5 centre (-129.159, 14.5859) radius 6
  line L7 (-146.963, 98.2669) -> (-43.681, 98.2669) projected
  circle A6 centre (-56.293, 14.5859) radius 6
  point P0 (0, 0)
  dimension "d102" = 12
  dimension "d103" = 83.789
  dimension "d104" = 19.949
  dimension "d107" = 12
  dimension "d108" = 93.567
  dimension "d109" = 154.737
  dimension "d110" = 12
  dimension "d111" = 85.478
  dimension "d112" = 83.833
  dimension "d113" = 12
  dimension "d114" = 12.612
  dimension "d115" = 83.833
  dimension "d116" = 12
  dimension "d117" = 17.092
  dimension "d118" = 83.833
  dimension "d119" = 12
  dimension "d120" = 85.478
  dimension "d121" = 83.681
  dimension "d122" = 12
  dimension "d123" = 12.612
  dimension "d124" = 83.681
  constraints: 7 centre point
  measures "d102" diameter of A0
  measures "d103" distance from line of L0 A0.centre
  measures "d104" distance from line of L1 A0.centre
  measures "d107" diameter of A1
  measures "d108" distance from line of L2 A1.centre
  measures "d109" distance from line of L1 A1.centre
  measures "d110" diameter of A2
  measures "d111" distance from line of L3 A2.centre
  measures "d112" distance from line of L4 A2.centre
  measures "d113" diameter of A3
  measures "d114" distance from line of L3 A3.centre
  measures "d115" distance from line of L4 A3.centre
  measures "d116" diameter of A4
  measures "d117" distance from line of L5 A4.centre
  measures "d118" distance from line of L6 A4.centre
  measures "d119" diameter of A5
  measures "d120" distance from line of L3 A5.centre
  measures "d121" distance from line of L7 A5.centre
  measures "d122" diameter of A6
  measures "d123" distance from line of L3 A6.centre
  measures "d124" distance from line of L7 A6.centre
extrude "Extrusion11" cut sketch "Sketch9" against normal up to surface (8.255 mm away)
fillet "Fillet4" radius 3 16 edges at (387.6295, 98.2669, -4.1275) (399.5103, 98.2669, -4.1275) (264.7024, 98.2669, -4.1275) (252.8615, 98.2669, -4.1275) (135.0683, 98.2669, -4.1275) (123.2497, 98.2669, -4.1275) (62.2023, 98.2669, -4.1275) (50.3837, 98.2669, -4.1275) (50.359, 15.4734, -4.1275) (62.227, 15.4734, -4.1275) (123.225, 15.4734, -4.1275) (135.093, 15.4734, -4.1275) (191.7214, 15.4734, -4.1275) (343.0651, 15.3216, -4.1275) (388.492, 15.3216, -4.1275) (400.36, 15.3216, -4.1275)
sketch "Sketch10" plane through (0, 0, 0) normal (0, 0, -1) x (-1, 0, 0)
  arc A0 (-387.7447, 100.5481) -> (-399.3952, 100.5481) centre (-393.5699, 99.1106) ccw projected
  arc A1 (-252.936, 100.5915) -> (-264.6279, 100.5915) centre (-258.7819, 99.2406) ccw projected
  arc A2 (-123.3031, 100.6134) -> (-135.0149, 100.6134) centre (-129.159, 99.3064) ccw projected
  arc A3 (-50.4371, 100.6134) -> (-62.1489, 100.6134) centre (-56.293, 99.3064) ccw projected
  arc A4 (-62.1254, 13.1776) -> (-50.4606, 13.1776) centre (-56.293, 14.5859) ccw projected
  arc A5 (-134.9914, 13.1776) -> (-123.3266, 13.1776) centre (-129.159, 14.5859) ccw projected
  arc A6 (-400.2584, 13.0257) -> (-388.5936, 13.0257) centre (-394.426, 14.4339) ccw projected
  line L0 (-267.5509, 98.2669) -> (-384.8321, 98.2669) projected
  line L1 (-343.0651, 12.3216) -> (-343.0651, 5.6736) projected
  point P0 (0, 0)
  point P1 (-266.6151, 12.9809)
  dimension "d128" = 85.286
  dimension "d129" = 76.45
  constraints: 7 coincident
  measures "d128" distance from line of L0 point (-266.615, 12.981)
  measures "d129" distance from line of L1 point (-266.615, 12.981)
hole "Hole1" at (393.5699, 99.1106, 0) at (258.7819, 99.2406, 0) at (129.159, 99.3064, 0) at (56.293, 99.3064, 0) at (56.293, 14.5859, 0) at (129.159, 14.5859, 0) at (394.426, 14.4339, 0) at (266.6151, 12.9809, 0) direction (0, 0, 1) diameter 3 depth 5
move faces "Move7" translate (2, 0, 0) faces at (416.518, 35.8714, -2.9533)
move faces "Move8" translate (-2, 0, 0) faces at (38.681, 35.8714, -2.9533)
sketch "Sketch12" plane through (0, 0, 0) normal (0, 0, -1) x (-1, 0, 0)
  line L0 (-191.7214, 5.6736) -> (-343.0651, 5.6736) projected
  line L1 (-343.0651, 12.3216) -> (-343.0651, 5.6736) projected
  line L2 (-265.7681, 8.6736) -> (-262.2681, 8.6736)
  line L3 (-265.7681, 8.6736) -> (-269.2681, 8.6736)
  line L4 (-269.2681, 8.6736) -> (-269.2681, 5.6736)
  line L5 (-343.0651, 5.6736) -> (-191.7214, 5.6736) projected
  line L6 (-262.2681, 8.6736) -> (-262.2681, 5.6736)
  point P0 (0, 0)
  dimension "d145" = 3.5
  dimension "d146" = 3.5
  constraints: 8 end point, 2 horizontal, 2 perpendicular, 2 point on line
  measures "d145" distance of L2.start L2.end
  measures "d146" distance of L2.start L3.end
extrude "Extrusion12" add sketch "Sketch12" along normal up to surface (8.255 mm away)
sketch "Sketch13" plane through (0, 0, -8.255) normal (0, 0, -1) x (-1, 0, 0)
  line L0 (-159.963, 106.2669) -> (-418.518, 106.2669) projected
  line L1 (-418.518, 106.2669) -> (-418.518, 0.6736) projected
  line L2 (-36.681, 106.2669) -> (-148.963, 106.2669) projected
  line L3 (-36.681, 0.6736) -> (-36.681, 106.2669) projected
  line L4 (-418.518, 0.6736) -> (-36.681, 0.6736) projected
  line L5 (-269.2681, 5.6736) -> (-269.2681, 8.6736) projected
  point P0 (0, 0)
  point P1 (-40.681, 7.6736)
  point P2 (-40.681, 102.2669)
  point P3 (-414.5252, 7.6736)
  point P4 (-414.518, 102.2669)
  point P5 (-39.5539, 54.3867)
  point P6 (-414.5252, 54.3867)
  point P7 (-265.7681, 4.6736)
  point P8 (-153.2146, 7.6736)
  point P9 (-350.8417, 7.6736)
  point P10 (-321.059, 102.2669)
  point P11 (-227.5995, 102.2669)
  point P12 (-140.5995, 102.2669)
  dimension "d149" = 4
  dimension "d150" = 4
  dimension "d151" = 4
  dimension "d152" = 4
  dimension "d153" = 4
  dimension "d154" = 4
  dimension "d155" = 7
  dimension "d156" = 7
  dimension "d157" = 4
  dimension "d158" = 7
  dimension "d159" = 7
  dimension "d160" = 186.9185
  dimension "d161" = 87
  dimension "d162" = 93.4595
  dimension "d163" = 4
  dimension "d164" = 4
  dimension "d165" = 3.5
  dimension "d166" = 112.5535
  measures "d149" distance from line of point (-414.518, 102.267) L0
  measures "d150" distance from line of L1 point (-414.518, 102.267)
  measures "d151" distance from line of point (-321.059, 102.267) L0
  measures "d152" distance from line of point (-40.681, 102.267) L2
  measures "d153" distance from line of L3 point (-40.681, 102.267)
  measures "d154" distance from line of L3 point (-40.681, 7.674)
  measures "d155" distance from line of L4 point (-40.681, 7.674)
  measures "d156" distance from line of L4 point (-153.215, 7.674)
  measures "d157" distance from line of L4 point (-265.768, 4.674)
  measures "d158" distance from line of L4 point (-350.842, 7.674)
  measures "d159" distance from line of L4 point (-414.525, 7.674)
  measures "d160" distance of point (-40.681, 102.267) point (-227.6, 102.267)
  measures "d161" distance of point (-140.6, 102.267) point (-227.6, 102.267)
  measures "d162" distance of point (-321.059, 102.267) point (-227.6, 102.267)
  measures "d163" distance from line of L0 point (-227.6, 102.267)
  measures "d164" distance from line of point (-140.6, 102.267) L2
  measures "d165" distance from line of L5 point (-265.768, 4.674)
  measures "d166" horizontal distance of point (-265.768, 4.674) point (-153.215, 7.674)
hole "Hole2" at (40.681, 7.6736, -8.255) at (40.681, 102.2669, -8.255) at (414.5252, 7.6736, -8.255) at (414.518, 102.2669, -8.255) at (39.5539, 54.3867, -8.255) at (414.5252, 54.3867, -8.255) at (265.7681, 4.6736, -8.255) at (153.2146, 7.6736, -8.255) at (350.8417, 7.6736, -8.255) at (321.059, 102.2669, -8.255) at (227.5995, 102.2669, -8.255) at (140.5995, 102.2669, -8.255) direction (0, 0, 1) diameter 3 depth 7
move faces "Move9" translate (0, 0, -0.7) faces at (240.3224, 1.5069, -8.255)
sketch "Sketch14" plane through (36.681, 106.2669, 7.65) normal (0, 1, 0) x (1, 0, 0)
  line L0 (114.282, 13.655) -> (121.282, 13.655) projected
  arc A0 (121.282, 13.655) -> (123.282, 15.655) centre (121.282, 15.655) ccw projected
  arc A1 (112.282, 15.655) -> (114.282, 13.655) centre (114.282, 15.655) ccw projected
  line L1 (123.282, 16.605) -> (123.282, 15.655) projected
  line L2 (112.282, 15.655) -> (112.282, 16.605) projected
  line L3 (125.282, 16.605) -> (125.282, 15.655)
  arc A2 (121.282, 11.655) -> (125.282, 15.655) centre (121.282, 15.655) ccw
  line L4 (121.282, 11.655) -> (114.282, 11.655)
  arc A3 (110.282, 15.655) -> (114.282, 11.655) centre (114.282, 15.655) ccw
  line L5 (110.282, 15.655) -> (110.282, 16.605)
  line L6 (123.282, 16.605) -> (381.837, 16.605) projected
  line L7 (0, 16.605) -> (112.282, 16.605) projected
  point P0 (-36.681, 7.65)
  dimension "d177" = 2
  constraints: 6 end point, 4 point on circle, 2 centre point, 4 other
  measures "d177" distance between parallel lines of L0 L4
extrude "Extrusion13" cut sketch "Sketch14" against normal blind 2
sketch "Sketch15" plane through (418.518, 0.6736, -8.955) normal (0, 0, -1) x (-1, 0, 0)
  line L0 (256.555, 105.5933) -> (0, 105.5933) projected
  line L1 (168.505, 97.5933) -> (256.555, 97.5933) projected
  line L2 (218.725, 105.5933) -> (228.725, 105.5933)
  line L3 (228.725, 105.5933) -> (228.725, 97.5933)
  line L4 (228.725, 97.5933) -> (218.725, 97.5933)
  line L5 (218.725, 97.5933) -> (218.725, 105.5933)
  line L6 (0, 105.5933) -> (0, 0) projected
  point P0 (418.518, -0.6736)
  point P1 (218.725, 97.5933)
  point P2 (228.725, 105.5933)
  dimension "d180" = 10
  dimension "d181" = 218.725
  constraints: 8 end point, 2 parallel, 2 point on line, 1 horizontal, 1 perpendicular
  measures "d180" distance of L3.end L4.end
  measures "d181" distance between parallel lines of L6 L5
extrude "Extrusion14" cut sketch "Sketch15" against normal blind 3
move faces "Move10" translate (-2, 0, 0) faces at (199.793, 103.6002, -7.955)
move faces "Move11" translate (2, 0, 0) faces at (189.793, 100.9336, -7.955)
move faces "Move12" translate (0, 0, -1.39) faces at (193.793, 100.9336, -5.955)
move faces "Move13" translate (0, 0, -0.805) faces at (195.793, 103.6002, -7.345)
sketch "Sketch16" plane through (36.681, 106.2669, 7.65) normal (0, 1, 0) x (1, 0, 0)
  line L0 (161.112, 15.8) -> (155.112, 15.8) projected
  line L1 (161.112, 16.605) -> (161.112, 15.8) projected
  line L2 (155.112, 15.8) -> (155.112, 16.605) projected
  line L3 (150.112, 16.605) -> (150.112, 10.8)
  line L4 (150.112, 10.8) -> (166.112, 10.8)
  line L5 (166.112, 10.8) -> (166.112, 16.605)
  line L6 (161.112, 16.605) -> (381.837, 16.605) projected
  line L7 (125.282, 16.605) -> (155.112, 16.605) projected
  point P0 (-36.681, 7.65)
  dimension "d196" = 5
  constraints: 6 end point, 2 other
  measures "d196" distance between parallel lines of L0 L4
extrude "Extrusion15" cut sketch "Sketch16" against normal blind 7
chamfer "Chamfer1" distance 3 angle 45 5 edges at (202.793, 106.2669, -8.15) (202.793, 106.2669, -5.2475) (194.793, 106.2669, -3.15) (186.793, 106.2669, -8.15) (186.793, 106.2669, -5.2475)
fillet "Fillet5" radius 5 8 edges at (36.681, 106.2669, -0.6525) (36.681, 0.6736, -0.6525) (418.518, 0.6736, -0.6525) (418.518, 106.2669, -0.6525) (418.518, 53.4702, 7.65) (227.5995, 106.2669, 7.65) (36.681, 53.4702, 7.65) (227.5995, 0.6736, 7.65)
chamfer "Chamfer2" distance 0.5 angle 45 43 edges at (85.4443, 95.8817, 7.65) (124.6706, 56.946, 7.65) (46.218, 56.946, 7.65) (85.4443, 18.0104, 7.65) (155.7315, 18.0104, 7.65) (180.093, 27.6298, 7.65) (187.8354, 36.1758, 7.65) (194.1461, 25.6701, 7.65) (131.37, 27.6298, 7.65) (129.274, 47.3247, 7.65) (130.322, 37.2493, 7.65) (130.75, 57.4, 7.65) (132.226, 67.0208, 7.65) (133.5125, 76.6415, 7.65) (134.799, 86.2616, 7.65) (154.9787, 95.8817, 7.65) (175.2203, 96.3218, 7.65) (213.5556, 91.3827, 7.65) (250.51, 76.5707, 7.65) (251.5424, 66.8074, 7.65) (252.5685, 57.0445, 7.65) (255.9585, 46.9489, 7.65) (257.947, 26.8766, 7.65) (224.02, 11.8527, 7.65) (307.1869, 12.1861, 7.65) (270.9016, 26.8777, 7.65) (272.8895, 46.95, 7.65) (276.356, 56.501, 7.65) (271.9135, 64.9398, 7.65) (274.2709, 65.2712, 7.65) (268.9885, 74.7023, 7.65) (306.8778, 90.2044, 7.65) (374.9084, 95.7299, 7.65) (403.647, 86.1098, 7.65) (406.314, 66.8689, 7.65) (408.981, 47.1728, 7.65) (407.6475, 57.2482, 7.65) (406.882, 27.478, 7.65) (382.5205, 17.8586, 7.65) (358.159, 27.478, 7.65) (352.8604, 37.0975, 7.65) (342.8274, 36.4321, 7.65) (339.4183, 26.3351, 7.65)
body "Solid3"
